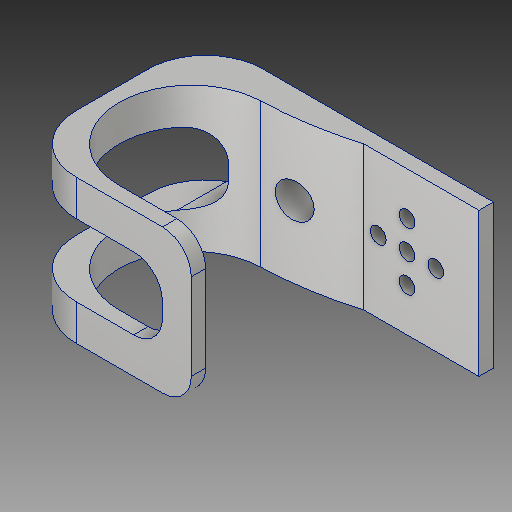
# Autodesk Inventor part: Maybe Hook
Saved by Autodesk Inventor 2019.4 (Build 234330000, 330)
## iProperties
Created: 2020-02-01
Part Number: Maybe Hook
Material: Aluminum 6061
Document SubType Name: Modeling
Designer: Mark
Mass: 131.55 g
Surface Area: 196.981 cm^2
Volume: 48.7224 cm^3
Density: 2.7 g/cm^3
Appearance: Aluminum - Flat
Author: Mark
Autodesk Inventor part; units mm, degrees
ref_plane "YZ Plane" through (0, 0, 0) normal (1, 0, 0) x (0, 1, 0)
ref_plane "XZ Plane" through (0, 0, 0) normal (0, 1, 0) x (-1, 0, 0)
ref_plane "XY Plane" through (0, 0, 0) normal (0, 0, 1) x (1, 0, 0)
sketch "Sketch1" plane through (0, 0, 0) normal (0, 1, 0) x (-1, 0, 0)
  line L0 (0, 0) -> (100, 0)
  line L1 (100, 0) -> (100, -5)
  line L2 (100, -5) -> (0, -5)
  line L3 (0, -5) -> (0, 0)
  circle A0 centre (70, 30) radius 25
  line L4 (40, 60) -> (100, 60)
  line L5 (100, 60) -> (100, 0)
  line L6 (100, 0) -> (40, 0)
  line L7 (40, 60) -> (100, 0) construction
  line L8 (100, 60) -> (40, 0) construction
  line L9 (70, 55) -> (40, 55)
  line L10 (70, 5) -> (40, 5)
  line L11 (40, 0) -> (40, 5)
  line L12 (40, 55) -> (40, 60)
  dimension "d0" = 100
  dimension "d1" = 5
  dimension "d2" = 50
  dimension "d3" = 30
  dimension "d4" = 30
  dimension "d5" = 60
  dimension "d6" = 60
  dimension "d8" = 60
  constraints: 26 end point, 6 perpendicular, 5 parallel, 2 horizontal, 2 midpoint, 2 point on circle, 2 tangent, 1 centre point
  measures "d0" distance of L1.end L2.end
  measures "d1" distance of L0.end L1.end
  measures "d2" diameter of A0
  measures "d3" distance from line of L1 A0.centre
  measures "d4" distance from line of L0 A0.centre
  measures "d5" distance of L5.end L6.end
  measures "d6" distance between parallel lines of L0 L4
  measures "d8" distance between parallel lines of L5 L12
extrude "Extrusion1" add sketch "Sketch1" along normal blind 50 contours L0 L1 L2 L3 | L11 L10 A0 L9 L12 L4 L5 L0
fillet "Fillet1" radius 122 1 edges at (-40, 25, 5)
fillet "Fillet2" radius 20 2 edges at (-100, 25, 60) (-100, 25, -5)
sketch "Sketch2" plane through (0, 0, 0) normal (0, 0, 1) x (1, 0, 0)
  circle A0 centre (-25, 25) radius 2.75
  circle A1 centre (-15, 25) radius 2.75
  circle A2 centre (-35, 25) radius 2.75
  circle A3 centre (-25, 15) radius 2.75
  circle A4 centre (-25, 35) radius 2.75
  line L0 (0, 0) -> (-40, 0) projected
  line L1 (0, 0) -> (0, 50) projected
  dimension "d13" = 5.5
  dimension "d14" = 5.5
  dimension "d15" = 5.5
  dimension "d16" = 5.5
  dimension "d17" = 5.5
  dimension "d18" = 10
  dimension "d19" = 25
  dimension "d20" = 25
  dimension "d21" = 25
  dimension "d22" = 20
  dimension "d23" = 10
  dimension "d24" = 15
  dimension "d25" = 10
  dimension "d26" = 10
  dimension "d27" = 10
  constraints: 5 centre point
  measures "d13" diameter of A0
  measures "d14" diameter of A1
  measures "d15" diameter of A2
  measures "d16" diameter of A3
  measures "d17" diameter of A4
  measures "d18" distance of A0.centre A4.centre
  measures "d19" distance from line of L0 A0.centre
  measures "d20" distance from line of L0 A2.centre
  measures "d21" distance from line of L0 A1.centre
  measures "d22" distance of A1.centre A2.centre
  measures "d23" distance of A2.centre A0.centre
  measures "d24" distance from line of L1 A1.centre
  measures "d25" distance of A0.centre A3.centre
  measures "d26" horizontal distance of A1.centre A4.centre
  measures "d27" horizontal distance of A1.centre A3.centre
extrude "Extrusion2" cut sketch "Sketch2" against normal blind 50
sketch "Sketch3" plane through (0, 0, -5) normal (0, 0, -1) x (-1, 0, 0)
  circle A0 centre (60, 25) radius 6
  line L0 (0, 0) -> (0, 50) projected
  line L1 (0, 50) -> (80, 50) projected
  dimension "d30" = 12
  dimension "d31" = 60
  dimension "d32" = 25
  constraints: 1 centre point
  measures "d30" diameter of A0
  measures "d31" distance from line of L0 A0.centre
  measures "d32" distance from line of L1 A0.centre
extrude "Extrusion3" cut sketch "Sketch3" against normal up to surface round surface about axis through (-74.8371, 0, -116.9204) along (0, 1, 0) radius 122 far side no
sketch "Sketch4" plane through (-100, 0, 15) normal (-1, 0, 0) x (0, 0, 1)
  line L0 (45, 37.5) -> (-20, 37.5)
  line L1 (-20, 37.5) -> (-20, 12.5)
  line L2 (-20, 12.5) -> (45, 12.5)
  line L3 (45, 12.5) -> (45, 37.5)
  line L4 (45, 37.5) -> (-20, 12.5) construction
  line L5 (-20, 37.5) -> (45, 12.5) construction
  line L6 (25, 0) -> (0, 0) projected
  line L7 (-20, 50) -> (-20, 0) projected
  line L8 (45, 0) -> (45, 50) projected
  point P0 (-15, 0)
  point P1 (12.5, 25)
  dimension "d36" = 25
  dimension "d37" = 12.5
  constraints: 12 end point, 2 collinear, 2 midpoint, 2 parallel, 1 horizontal, 1 perpendicular
  measures "d36" distance of L1.end L0.end
  measures "d37" distance between parallel lines of L6 L2
extrude "Extrusion4" cut sketch "Sketch4" against normal blind 20
sketch "Sketch5" plane through (-80, 0, 15) normal (-1, 0, 0) x (0, 0, 1)
  line L0 (37.9129, 12.5) -> (37.9129, 37.5) projected
  line L1 (45, 12.5) -> (37.9129, 12.5) projected
  line L2 (45, 12.5) -> (45, 37.5) projected
  line L3 (37.9129, 37.5) -> (45, 37.5) projected
  point P0 (-15, 0)
extrude "Extrusion5" cut sketch "Sketch5" against normal blind 30
fillet "Fillet3" radius 10 4 edges at (-50, 12.5, 57.5) (-50, 37.5, 57.5) (-80, 12.5, 1.0436) (-80, 37.5, 1.0436)
fillet "Fillet4" radius 10 2 edges at (-40, 50, 57.5) (-40, 0, 57.5)
body "Solid1"
